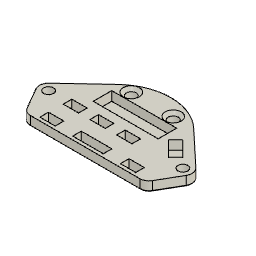
Toolhead Spacer (Autodesk Fusion 360 design; units mm, degrees)
Autodesk Fusion 360 part; units mm, degrees
sketch "Sketch1" plane through (0, 0, 0) normal (0, 0, 1) x (1, 0, 0)
  circle A0 centre (-0.7586, 1.4395) radius 1.025 construction
  circle A1 centre (2.2414, 1.4395) radius 1.025 construction
  circle A2 centre (5.2414, 1.4395) radius 0.55 construction
  circle A3 centre (-3.7586, 4.4395) radius 0.55 construction
  circle A4 centre (8.2414, 4.4395) radius 0.55 construction
  arc A5 (-23.5903, -2.1109) -> (-24.1355, -5.7985) centre (-21.5374, -4.2985) ccw
  arc A6 (18.2616, -14.2985) -> (20.8597, -12.7985) centre (18.2616, -11.2985) ccw
  circle A7 centre (-9.7586, 1.4395) radius 1.025 construction
  arc A8 (24.9006, -5.7985) -> (24.3555, -2.1109) centre (22.3026, -4.2984) ccw
  circle A9 centre (2.2414, 4.4395) radius 1.025 construction
  circle A10 centre (6.093, 8.7601) radius 1.625
  circle A11 centre (-6.7586, 1.4395) radius 1.025 construction
  circle A12 centre (5.2414, 4.4395) radius 1.025 construction
  circle A13 centre (5.2414, 4.4395) radius 0.55 construction
  circle A14 centre (22.3026, -4.2984) radius 1.6
  circle A15 centre (-3.7586, 1.4395) radius 1.025 construction
  circle A16 centre (-9.7586, 1.4395) radius 0.55 construction
  circle A17 centre (-9.7586, 4.4395) radius 0.55 construction
  circle A18 centre (-3.7586, 4.4395) radius 1.025 construction
  circle A19 centre (-7.6073, 8.7601) radius 1.625
  arc A20 (-20.094, -12.7985) -> (-17.4959, -14.2985) centre (-17.4959, -11.2985) ccw
  circle A21 centre (-3.7586, 1.4395) radius 0.55 construction
  arc A22 (12.7001, 8.827) -> (-11.9349, 8.827) centre (0.3826, -4.2985) ccw
  circle A23 centre (5.2414, 1.4395) radius 1.025 construction
  circle A24 centre (8.2414, 1.4395) radius 0.55 construction
  circle A25 centre (-0.7586, 4.4395) radius 0.55 construction
  circle A26 centre (-9.7586, 4.4395) radius 1.025 construction
  circle A27 centre (-11.7144, -11.8165) radius 0.5 construction
  line L0 (-15.1394, -10.8915) -> (-15.1394, -12.7415) construction
  line L1 (-6.2917, -5.2485) -> (-4.4417, -5.2485) construction
  line L2 (-13.2894, -10.8915) -> (-15.1394, -10.8915) construction
  circle A28 centre (-2.8667, -4.3235) radius 0.5 construction
  circle A29 centre (14.1746, 1.4296) radius 0.6 construction
  circle A30 centre (-3.5064, -11.8165) radius 0.5 construction
  circle A31 centre (-6.7586, 1.4395) radius 0.55 construction
  circle A32 centre (-6.7586, 4.4395) radius 1.025 construction
  circle A33 centre (-11.5874, -4.3235) radius 0.925 construction
  circle A34 centre (14.5746, -11.8165) radius 0.925 construction
  line L3 (-16.5874, -6.7235) -> (-16.5874, -0.9235) construction
  circle A35 centre (2.2414, 1.4395) radius 0.55 construction
  circle A36 centre (-21.5374, -4.2985) radius 1.6
  circle A37 centre (-11.5874, -4.3235) radius 0.5 construction
  circle A38 centre (8.2414, 4.4395) radius 1.025 construction
  circle A39 centre (2.2414, 4.4395) radius 0.55 construction
  circle A40 centre (8.2414, 1.4395) radius 1.025 construction
  circle A41 centre (-0.7586, 1.4395) radius 0.55 construction
  circle A42 centre (-2.8667, -4.3235) radius 0.925 construction
  circle A43 centre (-0.7586, 4.4395) radius 1.025 construction
  circle A44 centre (-6.7586, 4.4395) radius 0.55 construction
  line L4 (-9.0874, -0.9235) -> (-9.0874, -6.7235) construction
  circle A45 centre (3.9936, -11.8165) radius 0.5 construction
  circle A46 centre (14.5746, -11.8165) radius 0.5 construction
  line L5 (-13.2894, -12.7415) -> (-13.2894, -10.8915) construction
  line L6 (2.429, -5.2485) -> (4.2789, -5.2485) construction
  circle A47 centre (14.1746, 1.4296) radius 1.175 construction
  line L7 (-15.0124, -5.2485) -> (-13.1624, -5.2485) construction
  line L8 (-15.1394, -12.7415) -> (-13.2894, -12.7415) construction
  circle A48 centre (16.8687, -1.2645) radius 0.6 construction
  line L9 (2.429, -3.3985) -> (2.429, -5.2485) construction
  circle A49 centre (-1.0064, -11.8165) radius 0.5 construction
  line L10 (-13.1624, -5.2485) -> (-13.1624, -3.3985) construction
  line L11 (12.9996, -12.7415) -> (12.9996, -10.8915) construction
  circle A50 centre (-14.0874, -4.3235) radius 0.5 construction
  circle A51 centre (3.3539, -4.3235) radius 0.5 construction
  line L12 (-16.0925, -6.2285) -> (-16.0925, -1.4025) construction
  circle A52 centre (-5.3667, -4.3235) radius 0.5 construction
  line L13 (-13.1624, -3.3985) -> (-15.0124, -3.3985) construction
  line L14 (11.1496, -10.8915) -> (11.1496, -12.7415) construction
  line L15 (11.5936, -13.7215) -> (11.5936, -14.2165) construction
  line L16 (-7.8667, -0.9235) -> (-0.3667, -0.9235) construction
  circle A53 centre (-11.7144, -11.8165) radius 0.925 construction
  line L17 (-7.8667, -6.7235) -> (-0.3667, -6.7235) construction
  circle A54 centre (-1.0064, -11.8165) radius 0.925 construction
  circle A55 centre (1.4936, -11.8165) radius 0.925 construction
  line L18 (-10.9794, -6.2285) -> (-10.9794, -6.7235) construction
  line L19 (16.8687, 0.3972) -> (15.207, -1.2645) construction
  line L20 (-0.3667, -0.9235) -> (-0.3667, -6.7235) construction
  line L21 (-6.2917, -3.3985) -> (-6.2917, -5.2485) construction
  circle A56 centre (12.0746, -11.8165) radius 0.5 construction
  line L22 (-16.0925, -1.4025) -> (-9.7095, -1.4025) construction
  line L23 (-15.0124, -3.3985) -> (-15.0124, -5.2485) construction
  line L24 (1.3489, -6.2285) -> (1.3489, -1.4025) construction
  line L25 (10.0695, -13.7215) -> (10.0695, -8.8955) construction
  line L26 (-7.3718, -1.4025) -> (-0.9888, -1.4025) construction
  line L27 (-4.4417, -3.3985) -> (-6.2917, -3.3985) construction
  line L28 (9.5746, -8.4165) -> (17.0746, -8.4165) construction
  line L29 (-16.7144, -14.2165) -> (-9.2144, -14.2165) construction
  line L30 (-9.8365, -8.8955) -> (-9.8365, -13.7215) construction
  line L31 (1.3489, -1.4025) -> (7.7319, -1.4025) construction
  line L32 (18.5304, -1.2645) -> (16.8687, 0.3972) construction
  line L33 (-13.6794, -6.2285) -> (-13.6794, -6.7235) construction
  line L34 (4.2789, -3.3985) -> (2.429, -3.3985) construction
  line L35 (-2.2587, -6.2285) -> (-2.2587, -6.7235) construction
  line L36 (-9.7095, -1.4025) -> (-9.7095, -6.2285) construction
  circle A57 centre (3.9936, -11.8165) radius 0.925 construction
  circle A58 centre (5.8539, -4.3235) radius 0.925 construction
  line L37 (-4.4417, -5.2485) -> (-4.4417, -3.3985) construction
  circle A59 centre (5.8539, -4.3235) radius 0.5 construction
  line L38 (-9.7095, -6.2285) -> (-16.0925, -6.2285) construction
  line L39 (-16.5874, -0.9235) -> (-9.0874, -0.9235) construction
  line L40 (12.9996, -10.8915) -> (11.1496, -10.8915) construction
  line L41 (-11.9954, -6.2285) -> (-11.9954, -6.7235) construction
  circle A60 centre (1.4936, -11.8165) radius 0.5 construction
  line L42 (16.8687, -2.9262) -> (18.5304, -1.2645) construction
  line L43 (4.2789, -5.2485) -> (4.2789, -3.3985) construction
  line L44 (11.1496, -12.7415) -> (12.9996, -12.7415) construction
  line L45 (-14.5684, -6.2285) -> (-14.5684, -6.7235) construction
  circle A61 centre (-3.5064, -11.8165) radius 0.925 construction
  line L46 (15.1826, -13.7215) -> (15.1826, -14.2165) construction
  line L47 (15.207, -1.2645) -> (16.8687, -2.9262) construction
  line L48 (-0.9888, -1.4025) -> (-0.9888, -6.2285) construction
  line L49 (-16.5874, -6.7235) -> (-9.0874, -6.7235) construction
  circle A62 centre (-14.2144, -11.8165) radius 0.5 construction
  line L50 (6.4936, -14.2165) -> (6.4936, -8.4165) construction
  line L51 (7.7319, -1.4025) -> (7.7319, -6.2285) construction
  line L52 (11.5445, 13.4388) -> (-13.0519, 13.4388) construction
  line L53 (-16.7144, -8.4165) -> (-9.2144, -8.4165) construction
  line L54 (-7.3718, -6.2285) -> (-7.3718, -1.4025) construction
  line L55 (3.7619, -6.2285) -> (3.7619, -6.7235) construction
  line L56 (7.7319, -6.2285) -> (1.3489, -6.2285) construction
  line L57 (-13.8064, -13.7215) -> (-13.8064, -14.2165) construction
  line L58 (-13.0493, 2.9384) -> (11.5445, 2.9384) construction
  line L59 (-5.5115, -8.8955) -> (-5.5115, -13.7215) construction
  line L60 (11.5445, 2.9384) -> (11.5445, 13.4388) construction
  line L61 (-12.1224, -13.7215) -> (-12.1224, -14.2165) construction
  line L62 (-2.2557, 11.9395) -> (-2.2557, 13.4388) construction
  line L63 (14.1666, -13.7215) -> (14.1666, -14.2165) construction
  line L64 (-0.9888, -6.2285) -> (-7.3718, -6.2285) construction
  line L65 (-5.5115, -13.7215) -> (5.8715, -13.7215) construction
  line L66 (9.5746, -14.2165) -> (17.0746, -14.2165) construction
  line L67 (16.3856, -5.013) -> (10.431, 0.9417) construction
  line L68 (-9.8365, -13.7215) -> (-16.2195, -13.7215) construction
  line L69 (5.8715, -8.8955) -> (-5.5115, -8.8955) construction
  line L70 (0.7443, 13.4388) -> (0.7443, 11.9395) construction
  line L71 (8.3539, -0.9235) -> (8.3539, -6.7235) construction
  line L72 (2.8729, -6.2285) -> (2.8729, -6.7235) construction
  line L73 (5.8715, -13.7215) -> (5.8715, -8.8955) construction
  line L74 (12.4826, -13.7215) -> (12.4826, -14.2165) construction
  line L75 (-7.8667, -6.7235) -> (-7.8667, -0.9235) construction
  line L76 (9.5746, -14.2165) -> (9.5746, -8.4165) construction
  line L77 (-3.2747, -6.2285) -> (-3.2747, -6.7235) construction
  line L78 (-9.2144, -8.4165) -> (-9.2144, -14.2165) construction
  line L79 (6.4936, -8.4165) -> (-6.0064, -8.4165) construction
  line L80 (-13.0519, 13.4388) -> (-13.0493, 2.9384) construction
  line L81 (-16.7144, -14.2165) -> (-16.7144, -8.4165) construction
  line L82 (0.854, -6.7235) -> (8.3539, -6.7235) construction
  line L83 (-16.2195, -13.7215) -> (-16.2195, -8.8955) construction
  line L84 (10.0695, -8.8955) -> (16.4525, -8.8955) construction
  line L85 (5.4459, -6.2285) -> (5.4459, -6.7235) construction
  line L86 (16.4525, -8.8955) -> (16.4525, -13.7215) construction
  line L87 (-14.6954, -13.7215) -> (-14.6954, -14.2165) construction
  line L88 (0.854, -0.9235) -> (8.3539, -0.9235) construction
  line L89 (15.8895, 1.3311) -> (14.0848, 3.1358) construction
  line L90 (-11.1064, -13.7215) -> (-11.1064, -14.2165) construction
  line L91 (3.5856, -14.2165) -> (3.5856, -13.7215) construction
  line L92 (-3.0984, -14.2165) -> (-3.0984, -13.7215) construction
  line L93 (21.3355, -0.063) -> (16.3856, -5.013) construction
  line L94 (14.0848, 3.1358) -> (16.1107, 5.1618) construction
  line L95 (17.9154, 3.3571) -> (15.8895, 1.3311) construction
  line L96 (-6.0064, -8.4165) -> (-6.0064, -14.2165) construction
  line L97 (15.3753, 5.8971) -> (21.3355, -0.063) construction
  line L98 (18.4851, -1.2645) -> (16.7789, 0.4417) construction
  line L99 (16.4525, -13.7215) -> (10.0695, -13.7215) construction
  line L100 (-6.0064, -14.2165) -> (6.4936, -14.2165) construction
  line L101 (-4.9587, -6.2285) -> (-4.9587, -6.7235) construction
  line L102 (-3.9874, -14.2165) -> (-3.9874, -13.7215) construction
  line L103 (6.4619, -6.2285) -> (6.4619, -6.7235) construction
  line L104 (0.854, -6.7235) -> (0.854, -0.9235) construction
  line L105 (16.7789, 0.4417) -> (18.8048, 2.4677) construction
  line L106 (17.0746, -8.4165) -> (17.0746, -14.2165) construction
  line L107 (10.431, 0.9417) -> (15.3753, 5.8971) construction
  line L108 (20.5111, 0.7614) -> (18.4851, -1.2645) construction
  line L109 (4.6016, -14.2165) -> (4.6016, -13.7215) construction
  line L110 (-5.8477, -6.2285) -> (-5.8477, -6.7235) construction
  line L111 (0.7443, 11.9395) -> (-2.2557, 11.9395) construction
  line L112 (-16.2195, -8.8955) -> (-9.8365, -8.8955) construction
  line L113 (-24.1355, -5.7985) -> (-20.094, -12.7985)
  line L114 (-17.4959, -14.2985) -> (18.2616, -14.2985)
  line L115 (20.8597, -12.7985) -> (24.9006, -5.7985)
  line L116 (24.3555, -2.1109) -> (12.7001, 8.827)
  line L117 (-11.9349, 8.827) -> (-23.5903, -2.1109)
  line L118 (-11.2433, 6.0093) -> (9.9773, 6.0093)
  line L119 (9.9773, 6.0093) -> (9.9773, -0.024)
  line L120 (9.9773, -0.024) -> (-11.2433, -0.024)
  line L121 (-11.2433, -0.024) -> (-11.2433, 6.0093)
  line L122 (-15.3374, -2.9235) -> (-10.3374, -2.9235)
  line L123 (-10.3374, -2.9235) -> (-10.3374, -5.7235)
  line L124 (-10.3374, -5.7235) -> (-15.3374, -5.7235)
  line L125 (-15.3374, -5.7235) -> (-15.3374, -2.9235)
  line L126 (2.1039, -5.7235) -> (2.1039, -2.9235)
  line L127 (2.1039, -2.9235) -> (7.1039, -2.9235)
  line L128 (7.1039, -5.7235) -> (2.1039, -5.7235)
  line L129 (7.1039, -2.9235) -> (7.1039, -5.7235)
  line L130 (-15.4644, -13.2165) -> (-15.4644, -10.4165)
  line L131 (-15.4644, -10.4165) -> (-10.4644, -10.4165)
  line L132 (-10.4644, -13.2165) -> (-15.4644, -13.2165)
  line L133 (-10.4644, -10.4165) -> (-10.4644, -13.2165)
  line L134 (10.8246, -10.4165) -> (15.8246, -10.4165)
  line L135 (10.8246, -13.2165) -> (10.8246, -10.4165)
  line L136 (15.8246, -13.2165) -> (10.8246, -13.2165)
  line L137 (15.8246, -10.4165) -> (15.8246, -13.2165)
  line L138 (-12.8374, -5.7235) -> (-12.8374, -2.9235) construction
  line L139 (-12.8374, -5.7235) -> (-15.3374, -2.9235) construction
  line L140 (-6.6167, -2.9235) -> (-1.6167, -2.9235)
  line L141 (-1.6167, -2.9235) -> (-1.6167, -5.7235)
  line L142 (-1.6167, -5.7235) -> (-6.6167, -5.7235)
  line L143 (-6.6167, -5.7235) -> (-6.6167, -2.9235)
  line L144 (-4.1167, -5.7235) -> (-4.1167, -2.9235) construction
  line L145 (-6.6167, -2.9235) -> (-4.1167, -5.7235) construction
  line L146 (4.6039, -2.9235) -> (4.6039, -5.7235)
  line L147 (2.1039, -2.9235) -> (4.6039, -5.7235) construction
  line L148 (-12.9644, -10.4165) -> (-12.9644, -13.2165) construction
  line L149 (-12.9644, -13.2165) -> (-15.4644, -10.4165) construction
  line L150 (13.3246, -10.4165) -> (13.3246, -13.2165) construction
  line L151 (10.8246, -10.4165) -> (13.3246, -13.2165) construction
  line L152 (-4.7564, -10.4165) -> (5.2436, -10.4165)
  line L153 (5.2436, -10.4165) -> (5.2436, -13.2165)
  line L154 (5.2436, -13.2165) -> (-4.7564, -13.2165)
  line L155 (-4.7564, -13.2165) -> (-4.7564, -10.4165)
  line L156 (-1.0064, -11.8165) -> (1.4936, -11.8165) construction
  line L157 (0.2436, -13.2165) -> (0.2436, -10.4165) construction
  line L158 (11.9262, 1.3968) -> (16.8687, -3.5457)
  line L159 (16.8687, -3.5457) -> (19.1847, -1.2296)
  line L160 (19.1847, -1.2296) -> (14.2422, 3.7129)
  line L161 (11.9262, 1.3968) -> (14.2422, 3.7129)
  dimension "d1" = 2.8
  dimension "d2" = 5
  dimension "d3" = 10
  constraint tangent A20 L113
  constraint tangent A6 L114
  constraint tangent A22 L116
  constraint tangent A5 L117
  constraint horizontal L118
  constraint vertical L119
  constraint horizontal L120
  constraint vertical L121
  constraint horizontal L122
  constraint vertical L123
  constraint horizontal L124
  constraint vertical L125
  constraint horizontal L127
  constraint vertical L129
  constraint horizontal L128
  constraint vertical L126
  constraint horizontal L131
  constraint vertical L133
  constraint horizontal L132
  constraint vertical L130
  constraint horizontal L134
  constraint vertical L137
  constraint horizontal L136
  constraint vertical L135
  constraint midpoint L124 L138.start
  constraint midpoint L122 L138.end
  constraint midpoint A50.centre L139
  constraint horizontal L140
  constraint vertical L141
  constraint horizontal L142
  constraint vertical L143
  constraint midpoint L142 L144.start
  constraint midpoint L140 L144.end
  constraint midpoint L127 L146.start
  constraint midpoint L128 L146.end
  constraint midpoint L131 L148.start
  constraint midpoint L132 L148.end
  constraint parallel L147 L149
  constraint midpoint L134 L150.start
  constraint midpoint L136 L150.end
  constraint parallel L149 L151
  constraint midpoint A62.centre L149
  constraint midpoint A52.centre L145
  constraint midpoint A51.centre L147
  constraint midpoint A56.centre L151
  constraint equal L122 L140
  constraint equal L127 L140
  constraint equal L131 L140
  constraint equal L127 L134
  constraint equal L125 L143
  constraint equal L126 L141
  constraint horizontal L152
  constraint vertical L153
  constraint horizontal L154
  constraint vertical L155
  constraint equal L133 L155
  constraint coincident A49.centre A54.centre
  constraint coincident A55.centre A60.centre
  constraint midpoint L154 L157.start
  constraint midpoint L152 L157.end
  constraint midpoint L156 L157
  constraint perpendicular L42 L158
  constraint perpendicular L158 L159
  constraint perpendicular L94 L160
  constraint coincident L160 L161.end
  constraint perpendicular L160 L161
  constraint coincident L160.end L161.end
  measures "d1" distance of L122.start L124.end
  measures "d2" distance of L122.start L122.end
  measures "d3" distance of L152.start L152.end
extrude "Extrude1" add sketch "Sketch1" along normal blind 3.2
sketch "Sketch3" plane through (0, 0, 0) normal (0, 0, -1) x (1, 0, 0)
  line L0 (-11.2433, 0.024) -> (9.9773, 0.024) construction
  line L1 (9.9773, 0.024) -> (9.9773, -6.0093)
  line L2 (9.9773, -6.0093) -> (-11.2433, -6.0093)
  line L3 (-11.2433, -6.0093) -> (-11.2433, 0.024)
  line L4 (-4.7564, 13.2165) -> (5.2436, 13.2165) construction
  line L5 (5.2436, 13.2165) -> (5.2436, 10.4165)
  line L6 (5.2436, 10.4165) -> (-4.7564, 10.4165)
  line L7 (-4.7564, 10.4165) -> (-4.7564, 13.2165)
  line L8 (-6.6167, 5.7235) -> (-1.6167, 5.7235) construction
  line L9 (-1.6167, 5.7235) -> (-1.6167, 2.9235)
  line L10 (-1.6167, 2.9235) -> (-6.6167, 2.9235)
  line L11 (-6.6167, 2.9235) -> (-6.6167, 5.7235)
  line L12 (-15.3374, 5.7235) -> (-10.3374, 5.7235) construction
  line L13 (-10.3374, 5.7235) -> (-10.3374, 2.9235)
  line L14 (-10.3374, 2.9235) -> (-15.3374, 2.9235)
  line L15 (-15.3374, 2.9235) -> (-15.3374, 5.7235)
  line L16 (16.8687, 3.5457) -> (19.1847, 1.2296)
  line L17 (19.1847, 1.2296) -> (14.2422, -3.7129)
  line L18 (14.2422, -3.7129) -> (11.9262, -1.3968)
  line L19 (11.9262, -1.3968) -> (16.8687, 3.5457) construction
  line L20 (7.1039, 2.9235) -> (2.1039, 2.9235)
  line L21 (2.1039, 2.9235) -> (2.1039, 5.7235)
  line L22 (2.1039, 5.7235) -> (7.1039, 5.7235) construction
  line L23 (7.1039, 5.7235) -> (7.1039, 2.9235)
  circle A0 centre (-7.6073, -8.7601) radius 1.625
  circle A1 centre (-21.5374, 4.2985) radius 1.6
  line L24 (-10.4644, 10.4165) -> (-15.4644, 10.4165)
  line L25 (-15.4644, 10.4165) -> (-15.4644, 13.2165)
  line L26 (-15.4644, 13.2165) -> (-10.4644, 13.2165) construction
  line L27 (-10.4644, 13.2165) -> (-10.4644, 10.4165)
  circle A2 centre (6.093, -8.7601) radius 1.625
  circle A3 centre (22.3026, 4.2984) radius 1.6
  line L28 (15.8246, 10.4165) -> (10.8246, 10.4165)
  line L29 (10.8246, 10.4165) -> (10.8246, 13.2165)
  line L30 (10.8246, 13.2165) -> (15.8246, 13.2165) construction
  line L31 (15.8246, 13.2165) -> (15.8246, 10.4165)
  line L32 (-23.5903, 2.1109) -> (-11.9349, -8.827)
  arc A4 (-11.9349, -8.827) -> (12.7001, -8.827) centre (0.3826, 4.2985) ccw
  line L33 (12.7001, -8.827) -> (24.3555, 2.1109)
  arc A5 (24.3555, 2.1109) -> (24.9006, 5.7985) centre (22.3026, 4.2984) ccw
  line L34 (24.9006, 5.7985) -> (20.8597, 12.7985)
  arc A6 (20.8597, 12.7985) -> (18.2616, 14.2985) centre (18.2616, 11.2985) ccw
  line L35 (18.2616, 14.2985) -> (-17.4959, 14.2985)
  arc A7 (-17.4959, 14.2985) -> (-20.094, 12.7985) centre (-17.4959, 11.2985) ccw
  line L36 (-20.094, 12.7985) -> (-24.1355, 5.7985)
  arc A8 (-24.1355, 5.7985) -> (-23.5903, 2.1109) centre (-21.5374, 4.2985) ccw
extrude "Extrude2" add sketch "Sketch3" against normal blind 0.2
chamfer "Chamfer1" distance 1 angle 45 2 edges at (-9.1223, 9.3477, 3.2) (4.578, 9.3477, 3.2)
chamfer "Chamfer2" distance 0.4 angle 45 10 edges at (0.3826, 13.7015, 0) (-17.7626, 3.3581, 0) (-24.5051, -3.8597, 0) (-22.1147, -9.2985, 0) (-18.9959, -13.8965, 0) (0.3828, -14.2985, 0) (19.7616, -13.8965, 0) (22.8801, -9.2985, 0) (25.2703, -3.8597, 0) (18.5278, 3.3581, 0)
